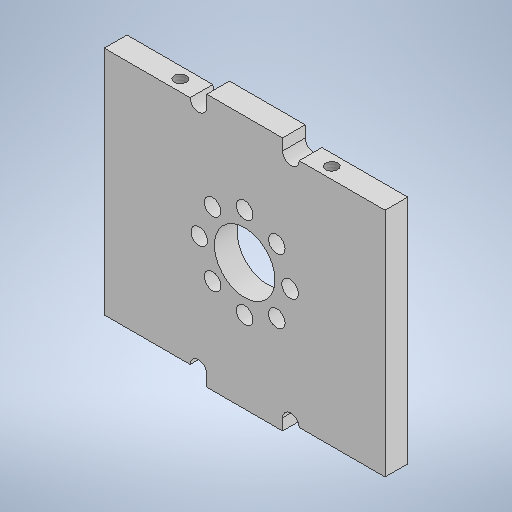
# Autodesk Inventor part: kosi_sita
Saved by Autodesk Inventor 2025.1 (Build 291241000, 241)
## iProperties
Created: 2024-08-31
Part Number: kosi_sita
Material: 一般
Document SubType Name: Modeling
Designer: right
Density: 1 g/cm^3
Appearance: 既定
Author: right
Autodesk Inventor part; units mm, degrees
ref_plane "YZ Plane" through (0, 0, 0) normal (1, 0, 0) x (0, 1, 0)
ref_plane "XZ Plane" through (0, 0, 0) normal (0, 1, 0) x (-1, 0, 0)
ref_plane "XY Plane" through (0, 0, 0) normal (0, 0, 1) x (1, 0, 0)
sketch "スケッチ1" plane through (0, 0, 0) normal (0, 0, 1) x (1, 0, 0)
  circle A0 centre (0, 0) radius 4
  circle A1 centre (0, 0) radius 6 construction
  circle A2 centre (0, 6) radius 1.1
  circle A3 centre (-4.2426, 4.2426) radius 1.1
  circle A4 centre (-6, 0) radius 1.1
  circle A5 centre (-4.2426, -4.2426) radius 1.1
  circle A6 centre (0, -6) radius 1.1
  circle A7 centre (4.2426, -4.2426) radius 1.1
  circle A8 centre (6, 0) radius 1.1
  circle A9 centre (4.2426, 4.2426) radius 1.1
  line L0 (-18.5321, -15.25) -> (18.5321, -15.25)
  line L1 (18.5321, -15.25) -> (18.5321, 15.25)
  line L2 (18.5321, 15.25) -> (-18.5321, 15.25)
  line L3 (-18.5321, 15.25) -> (-18.5321, -15.25)
  line L4 (-18.5321, -15.25) -> (18.5321, 15.25) construction
  line L5 (18.5321, -15.25) -> (-18.5321, 15.25) construction
  circle A10 centre (0, 0) radius 24
  line L6 (18.5321, 0) -> (-18.5321, 0) construction
  line L7 (0, 18.25) -> (0, 0) construction
  line L8 (-5, 15.25) -> (5, 15.25)
  line L9 (5, 15.25) -> (5, 16.75)
  line L10 (5, 16.75) -> (-5, 16.75)
  line L11 (-5, 16.75) -> (-5, 15.25)
  circle A11 centre (-6.1, 15.25) radius 1.1
  circle A12 centre (6.1, 15.25) radius 1.1
  line L12 (-5, -15.25) -> (5, -15.25)
  line L13 (5, -15.25) -> (5, -16.75)
  line L14 (5, -16.75) -> (-5, -16.75)
  line L15 (-5, -16.75) -> (-5, -15.25)
  circle A13 centre (-6.1, -15.25) radius 1.1
  circle A14 centre (6.1, -15.25) radius 1.1
  point P0 (0, 16.75)
  point P1 (0, -18.25)
  point P2 (0, -16.75)
  point P3 (7.2, 15.25)
  point P4 (-7.2, 15.25)
  point P5 (7.2, -15.25)
  point P6 (-7.2, -15.25)
  dimension "d1" = 12
  dimension "d11" = 48
  dimension "d23" = 2.2
  dimension "d24" = 2.2
  dimension "d0" = 8
  dimension "d2" = 2.2
  dimension "d5" = 360
  dimension "d20" = 30.5
  dimension "d21" = 1.5
  dimension "d22" = 10
  constraints: 32 end point, 9 centre point, 8 symmetric about line, 6 midpoint, 4 horizontal, 4 parallel, 4 vertical alignment, 3 coincident, 3 point on line, 2 perpendicular, 34 other
  measures "d0" diameter of A0
  measures "d2" diameter of A2
  measures "d20" distance between parallel lines of L0 L2
  measures "d21" distance between parallel lines of L2 L10
  measures "d22" distance between parallel lines of L9 L11
extrude "押し出し1" add sketch "スケッチ1" along normal blind 3 contours A13 L0 L3 L2 A11 A12 L1 A14 | L0 L13 L14 L15 | L0 A13 | A14 L0 | L2 A11 | A12 L2 | L11 L10 L9 L2 picked at (-6.0558, -14.886) picked at (6.1442, -14.886) picked at (-6.1442, 14.886) picked at (6.0558, 14.886)
extrude "押し出し2" cut sketch "スケッチ1" along normal blind 3 contours L0 A13 | A14 L0 | L2 A11 | A12 L2 picked at (-6.0558, -14.886) picked at (6.1442, -14.886) picked at (-6.1442, 14.886) picked at (6.0558, 14.886)
sketch "スケッチ2" plane through (18.5321, 15.25, 3) normal (0, 1, 0) x (1, 0, 0)
  line L0 (-13.5321, 3) -> (-13.5321, 0) projected
  line L1 (-23.5321, 3) -> (-23.5321, 0) projected
  point P0 (-18.5321, 3)
  point P1 (-8.5321, 1.5)
  point P2 (-28.5321, 1.5)
  point P3 (-13.5321, 1.5)
  point P4 (-23.5321, 1.5)
  dimension "d27" = 5
  dimension "d28" = 5
  constraints: 2 horizontal alignment, 2 midpoint
  measures "d27" distance from line of L0 point (-8.532, 1.5)
  measures "d28" distance from line of L1 point (-28.532, 1.5)
hole "穴1" at (10, 15.25, 1.5) at (-10, 15.25, 1.5) direction (0, -1, 0) diameter 1.567 end through all thread size "M2x0.4" class "6H" standard "ISO Metric profile"
equation "\"d28\" = d27"
